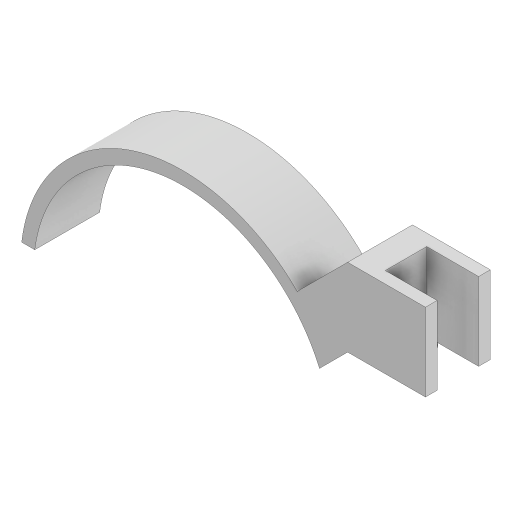
# Autodesk Inventor part: SOPORTE DE SENSOR INFRARROJO
Saved by Autodesk Inventor 2024 (Build 280153000, 153)
## iProperties
Created: 2024-07-05
Part Number: SOPORTE DE SENSOR INFRARROJO
Material: Generic
Document SubType Name: Modeling
Designer: Jhuliams
Density: 1 g/cm^3
Appearance: Default
Author: Jhuliams
Autodesk Inventor part; units mm, degrees
ref_plane "YZ Plane" through (0, 0, 0) normal (1, 0, 0) x (0, 1, 0)
ref_plane "XZ Plane" through (0, 0, 0) normal (0, 1, 0) x (-1, 0, 0)
ref_plane "XY Plane" through (0, 0, 0) normal (0, 0, 1) x (1, 0, 0)
sketch "Sketch3" plane through (0, 0, 0) normal (0, 0, 1) x (1, 0, 0)
  circle A0 centre (0, 0) radius 57.5
  arc A1 (44.1942, 44.1942) -> (56.5707, 26.5707) centre (0, 0) ccw
  line L0 (0, 0) -> (90, 0) construction
  line L1 (63.6396, 63.6396) -> (93.6396, 63.6396)
  line L2 (93.6396, 63.6396) -> (93.6396, 33.6396)
  line L3 (93.6396, 33.6396) -> (63.6396, 33.6396)
  line L4 (63.6396, 33.6396) -> (45, 15)
  line L5 (63.6396, 33.6396) -> (90, 33.6396) construction
  line L6 (-77.5, 7.5) -> (-47.5, 7.5)
  line L7 (-47.5, 7.5) -> (-47.5, -7.5)
  line L8 (-47.5, -7.5) -> (-77.5, -7.5)
  line L9 (-77.5, -7.5) -> (-77.5, 7.5)
  line L10 (-77.5, 7.5) -> (-47.5, -7.5) construction
  line L11 (-47.5, 7.5) -> (-77.5, -7.5) construction
  line L12 (0, 0) -> (40.6586, 40.6586)
  line L13 (44.1942, 44.1942) -> (63.6396, 63.6396)
  point P0 (-62.5, 0)
  point P1 (-62.0484, 7.5)
  point P2 (-57.0088, 7.5)
  point P3 (52.7905, 22.7905)
  dimension "d11" = 115
  dimension "d12" = 125
  dimension "d13" = 90
  dimension "d15" = 30
  dimension "d16" = 30
  dimension "d17" = 30
  dimension "d18" = 90
  dimension "d19" = 135
  dimension "d20" = 30
  dimension "d21" = 15
  constraints: 28 end point, 4 horizontal, 3 perpendicular, 3 point on circle, 2 coincident, 2 midpoint, 2 parallel, 1 centre point, 1 equal length, 1 point on line, 3 other
  measures "d12" diameter of A1
  measures "d13" distance of L0.start L1.start
  measures "d15" distance of L1.start L1.end
  measures "d16" distance of L1.end L2.end
  measures "d17" distance of L2.end L3.end
  measures "d18" angle of L2 L3
  measures "d19" angle of L4 L5
  measures "d20" distance of L7.end L8.end
  measures "d21" distance of L6.end L7.end
extrude "Extrusion3" add sketch "Sketch3" against normal blind 25 contours A0 L6 A1 L13 L1 L2 L3 L4
sketch "Sketch4" plane through (93.6396, 33.6396, 0) normal (1, 0, 0) x (0, 0, -1)
  line L0 (0, 0) -> (0, 30) projected
  line L1 (0, 0) -> (25, 0) projected
  line L2 (25, 30) -> (25, 0) projected
  line L3 (0, 30) -> (25, 30) projected
  line L4 (0, 0) -> (12.5, 0)
  line L5 (0, 0) -> (25, 0) projected
  line L6 (12.5, 0) -> (12.5, 15)
  line L7 (4.5, 40) -> (20.5, 40)
  line L8 (20.5, 40) -> (20.5, -10)
  line L9 (20.5, -10) -> (4.5, -10)
  line L10 (4.5, -10) -> (4.5, 40)
  line L11 (4.5, 40) -> (20.5, -10) construction
  line L12 (20.5, 40) -> (4.5, -10) construction
  point P0 (0, -33.6396)
  dimension "d24" = 12.5
  dimension "d25" = 15
  dimension "d26" = 16
  dimension "d27" = 50
  constraints: 16 end point, 3 midpoint, 2 parallel, 2 perpendicular, 1 horizontal
  measures "d24" distance of L0.start L4.end
  measures "d25" distance of L4.end L6.end
  measures "d26" distance of L8.end L9.end
  measures "d27" distance of L7.end L8.end
extrude "Extrusion4" cut sketch "Sketch4" against normal blind 20 contours L10 L3 L8 L1 | L1 L8 L9 L10 | L10 L7 L8 L3
sketch "Sketch5" plane through (73.6396, 33.6396, 0) normal (1, 0, 0) x (0, 0, -1)
  line L0 (4.5, 30) -> (20.5, 30) projected
  line L1 (4.5, 0) -> (4.5, 30) projected
  line L2 (20.5, 0) -> (4.5, 0) projected
  line L3 (20.5, 30) -> (20.5, 0) projected
  line L4 (12.5, 30) -> (12.5, 5)
  circle A0 centre (12.5, 5) radius 2.25
  point P0 (0, -33.6396)
  dimension "d30" = 25
  dimension "d31" = 4.5
  constraints: 2 end point, 1 centre point, 1 coincident, 1 midpoint, 1 vertical
  measures "d30" distance of L4.start L4.end
  measures "d31" diameter of A0
extrude "Extrusion5" add sketch "Sketch5" along normal blind 10 contours A0
fillet "Fillet1" radius 2 1 edges at (73.6396, 38.6396, -10.25)
body "Solid2"
